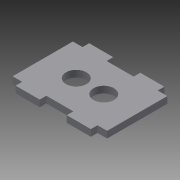
# Autodesk Inventor part: lado
Saved by Autodesk Inventor 2015 (Build 190159000, 159)
## iProperties
Created: 2017-11-28
Part Number: lado
Material: Generic
Document SubType Name: Modeling
Designer: Max
Density: 1 g/cm^3
Appearance: Default
Author: Max
Autodesk Inventor part; units mm, degrees
ref_plane "YZ Plane" through (0, 0, 0) normal (1, 0, 0) x (0, 1, 0)
ref_plane "XZ Plane" through (0, 0, 0) normal (0, 1, 0) x (-1, 0, 0)
ref_plane "XY Plane" through (0, 0, 0) normal (0, 0, 1) x (1, 0, 0)
sketch "Sketch1" plane through (0, 0, 0) normal (0, 0, 1) x (1, 0, 0)
  line L0 (-12.089, 0) -> (-12.089, -5.5)
  line L1 (-12.089, -5.5) -> (-32.089, -5.5)
  line L2 (-32.089, -5.5) -> (-32.089, 0)
  line L3 (-54.514, 0) -> (-54.514, -5.5)
  line L4 (-54.514, -5.5) -> (-74.514, -5.5)
  line L5 (-74.514, -5.5) -> (-74.514, 0)
  line L6 (-32.089, 0) -> (-54.514, 0)
  line L7 (-12.089, 50) -> (-12.089, 55.5)
  line L8 (-12.089, 55.5) -> (-32.089, 55.5)
  line L9 (-32.089, 55.5) -> (-32.089, 50)
  line L10 (-54.514, 50) -> (-54.514, 55.5)
  line L11 (-54.514, 55.5) -> (-74.514, 55.5)
  line L12 (-74.514, 55.5) -> (-74.514, 50)
  line L13 (-32.089, 50) -> (-54.514, 50)
  line L14 (-12.089, 0) -> (-4.089, 0)
  line L15 (-4.089, 0) -> (-4.089, 50)
  line L16 (-4.089, 50) -> (-12.089, 50)
  line L17 (-74.514, 50) -> (-82.514, 50)
  line L18 (-82.514, 50) -> (-82.514, 0)
  line L19 (-82.514, 0) -> (-74.514, 0)
  circle A0 centre (-31.877, 25) radius 8.5
  circle A1 centre (-54.726, 25) radius 8.5
  dimension "d2" = 5.5
  dimension "d3" = 20
  dimension "d4" = 5.5
  dimension "d5" = 20
  dimension "d6" = 90
  dimension "d18" = 8
  dimension "d20" = 8
  dimension "d22" = 17
  constraints: 40 end point, 8 perpendicular, 3 horizontal, 2 centre point, 1 vertical
  measures "d2" distance of L0.start L0.end
  measures "d3" distance of L0.end L1.end
  measures "d4" distance of L3.start L3.end
  measures "d5" distance of L3.end L4.end
  measures "d6" angle of L3 L4
  measures "d18" distance of L0.start L14.end
  measures "d20" distance of L12.end L17.end
  measures "d22" diameter of A0
extrude "Extrusion1" add sketch "Sketch1" along normal blind 5.5 contours L0 L1 L2 L6 L3 L4 L5 L19 L18 L17 L12 L11 L10 L13 L9 L8 L7 L16 L15 L14 | A0 | A1
sketch "Sketch3" plane through (0, 0, 5.5) normal (0, 0, 1) x (1, 0, 0)
  circle A0 centre (-31.877, 25) radius 8.5
  circle A1 centre (-54.726, 25) radius 8.5
  point P0 (0, 0)
  dimension "d23" = 17
  constraints: 2 centre point
  measures "d23" diameter of A0
extrude "Extrusion2" cut sketch "Sketch3" against normal blind 10
body "Solid1"
